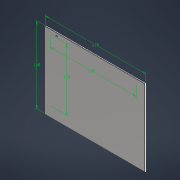
# Autodesk Inventor part: BackCover
Saved by Autodesk Inventor 2022 (Build 260153070, 153G)
## iProperties
Created: 2021-11-23
Part Number: BackCover
Material: Типовые
Document SubType Name: Обычные детали
Designer: kalugin_a
Density: 1 g/cm^3
Appearance: Нержавеющая — шлифованная
Author: kalugin_a
Autodesk Inventor part; units mm, degrees
ref_plane "YZ Plane" through (0, 0, 0) normal (1, 0, 0) x (0, 1, 0)
ref_plane "XZ Plane" through (0, 0, 0) normal (0, 1, 0) x (-1, 0, 0)
ref_plane "XY Plane" through (0, 0, 0) normal (0, 0, 1) x (1, 0, 0)
sketch "Эскиз1" plane through (0, 0, 0) normal (0, 0, 1) x (1, 0, 0)
  line L0 (0, 0) -> (-218, 0)
  line L1 (-218, 0) -> (-218, 166)
  line L2 (-218, 166) -> (0, 166)
  line L3 (0, 166) -> (0, 0)
  line L4 (-206.585, 154.4751) -> (-20.585, 154.4751)
  line L5 (-20.585, 154.4751) -> (-20.585, 20.4751)
  line L6 (-20.585, 20.4751) -> (-206.585, 20.4751)
  line L7 (-206.585, 20.4751) -> (-206.585, 154.4751)
  dimension "d0" = 218
  dimension "d1" = 166
  dimension "d7" = 186
  dimension "d8" = 134
  constraints: 16 end point, 4 parallel, 2 horizontal, 2 perpendicular
  measures "d0" distance of L1.end L2.end
  measures "d1" distance of L0.end L1.end
  measures "d7" distance of L4.start L4.end
  measures "d8" distance of L6.end L4.start
extrude "Выдавливание1" add sketch "Эскиз1" along normal blind 1.5 contours L0 L1 L2 L3 | L4 L5 L6 L7
chamfer "Фаска1" distance 0.3 angle 45 8 edges at (-109, 166, 1.5) (-218, 83, 1.5) (-109, 0, 1.5) (0, 83, 1.5) (-109, 166, 0) (0, 83, 0) (-218, 83, 0) (-109, 0, 0)
sketch "Эскиз2" plane through (0, 0, 1.5) normal (0, 0, 1) x (1, 0, 0)
  point P0 (0, 0)
  point P1 (-192.1806, 159.6518)
hole "Отверстие1" at (-192.1806, 159.6518, 1.5) direction (0, 0, -1) diameter 3 end through all countersink diameter 4 countersink angle 90
equation "\"Радиус_гибки\" = Толщина"
equation "\"Ширина_просечки\" = Толщина"
equation "\"Глубина_просечки\" = 0.5 * Толщина"
equation "\"Размер_просечки\" = 4 * Толщина"
equation "\"Мин_остаток\" = 2 * Толщина"
equation "\"Радиус_перехода\" = Радиус_гибки"
equation "\"Радиус_Якоби\" = Радиус_гибки"
equation "\"Размер_зазора\" = Толщина"
equation "\"Толщина\" = 3.048"
